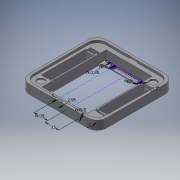
# Autodesk Inventor part: Bauteil1
Saved by Autodesk Inventor 2016 SP2 (Build 200236200, 236)
## iProperties
Created: 2018-06-26
Part Number: Bauteil1
Material: Generisch
Document SubType Name: Modeling
Designer: Nils
Density: 1 g/cm^3
Appearance: Vorgabe
Author: Nils
Autodesk Inventor part; units mm, degrees
ref_plane "YZ Plane" through (0, 0, 0) normal (1, 0, 0) x (0, 1, 0)
ref_plane "XZ Plane" through (0, 0, 0) normal (0, 1, 0) x (-1, 0, 0)
ref_plane "XY Plane" through (0, 0, 0) normal (0, 0, 1) x (1, 0, 0)
sketch "Skizze1" plane through (0, 0, 0) normal (0, 0, 1) x (1, 0, 0)
  line L0 (0, 0) -> (50.3, 0)
  line L1 (50.3, 0) -> (50.3, 70.3)
  line L2 (50.3, 70.3) -> (0, 70.3)
  line L3 (0, 70.3) -> (0, 0)
  line L4 (-15, 75.3) -> (65.3, 75.3)
  line L5 (65.3, 75.3) -> (65.3, -5)
  line L6 (65.3, -5) -> (-15, -5)
  line L7 (-15, -5) -> (-15, 75.3)
  line L8 (-11.7, 59.3) -> (-1.2, 59.3)
  line L9 (-1.2, 59.3) -> (-1.2, 11)
  line L10 (-1.2, 11) -> (-11.7, 11)
  line L11 (-11.7, 11) -> (-11.7, 59.3)
  line L12 (51.5, 59.3) -> (62, 59.3)
  line L13 (62, 59.3) -> (62, 11)
  line L14 (62, 11) -> (51.5, 11)
  line L15 (51.5, 11) -> (51.5, 59.3)
  line L16 (-6.45, 59.3) -> (-6.45, 75.3) construction
  line L17 (-6.45, 11) -> (-6.45, -5) construction
  line L18 (56.75, 59.3) -> (56.75, 75.3) construction
  line L19 (56.75, 11) -> (56.75, -5) construction
  line L20 (-11.7, 35.15) -> (-15, 35.15) construction
  line L21 (62, 35.15) -> (65.3, 35.15) construction
  line L22 (-8.4023, 11) -> (-1.7, 13)
  line L23 (-1.7, 13) -> (-4.95, 14.8)
  line L24 (-4.95, 14.8) -> (-7.95, 14.8)
  line L25 (-7.95, 14.8) -> (-7.95, 14)
  line L26 (-7.95, 14) -> (-5.1567, 14)
  line L27 (-5.1567, 14) -> (-3.7526, 13.2223)
  line L28 (-3.7526, 13.2223) -> (-11.2, 11)
  line L29 (58.25, 55.5) -> (55.25, 55.5)
  line L30 (55.25, 55.5) -> (55.25, 56.3)
  line L31 (55.25, 56.3) -> (58.0433, 56.3)
  line L32 (61.5, 57.3) -> (54.7977, 59.3)
  line L33 (59.4474, 57.0777) -> (52, 59.3)
  line L34 (58.0433, 56.3) -> (59.4474, 57.0777)
  line L35 (58.25, 55.5) -> (61.5, 57.3)
  line L36 (-10.7, 60.9) -> (-2.2, 60.9)
  line L37 (-2.2, 60.9) -> (-2.2, 63.9)
  line L38 (-2.2, 63.9) -> (-10.7, 63.9)
  line L39 (-10.7, 63.9) -> (-10.7, 60.9)
  line L40 (61, 6.4) -> (52.5, 6.4)
  line L41 (52.5, 6.4) -> (52.5, 9.4)
  line L42 (52.5, 9.4) -> (61, 9.4)
  line L43 (61, 9.4) -> (61, 6.4)
  dimension "d0" = 50.3
  dimension "d1" = 70.3
  dimension "d2" = 5
  dimension "d3" = 5
  dimension "d4" = 10.5
  dimension "d5" = 10.5
  dimension "d6" = 48.3
  dimension "d7" = 48.3
  dimension "d8" = 1.2
  dimension "d9" = 1.2
  dimension "d11" = 0.8
  dimension "d12" = 0.8
  dimension "d13" = 0.8
  dimension "d14" = 3
  dimension "d15" = 3.75
  dimension "d16" = 2
  dimension "d17" = 3
  dimension "d18" = 0.5
  dimension "d19" = 0.5
  dimension "d20" = 0.8
  dimension "d22" = 0.5
  dimension "d23" = 3
  dimension "d26" = 3.75
  dimension "d27" = 2
  dimension "d28" = 0.5
  dimension "d30" = 3
  dimension "d31" = 0.8
  dimension "d32" = 0.8
  dimension "d33" = 1.6
  dimension "d34" = 1
  dimension "d35" = 1
  dimension "d36" = 3
  dimension "d37" = 3
  dimension "d38" = 1
  dimension "d39" = 1
  dimension "d40" = 1.6
  constraints: 88 end point, 17 parallel, 13 perpendicular, 10 point on line, 8 midpoint, 7 horizontal, 4 equal length
  measures "d0" distance of L2.end L1.end
  measures "d1" distance of L1.end L0.end
  measures "d2" distance between parallel lines of L2 L4
  measures "d3" distance between parallel lines of L6 L0
  measures "d4" distance between parallel lines of L9 L11
  measures "d5" distance of L12.start L12.end
  measures "d6" distance between parallel lines of L10 L8
  measures "d7" distance of L12.end L13.end
  measures "d8" distance between parallel lines of L3 L9
  measures "d9" distance between parallel lines of L15 L1
  measures "d11" distance between parallel lines of L22 L28
  measures "d12" distance between parallel lines of L23 L27
  measures "d13" distance between parallel lines of L26 L24
  measures "d14" distance of L23.end L24.end
  measures "d15" distance between parallel lines of L11 L25
  measures "d16" distance from line of L10 L22.end
  measures "d17" distance between parallel lines of L10 L26
  measures "d18" distance of L28.end L10.end
  measures "d19" distance from line of L9 L22.end
  measures "d20" distance between parallel lines of L29 L31
  measures "d22" distance from line of L13 L32.start
  measures "d23" distance of L29.start L29.end
  measures "d26" distance between parallel lines of L15 L30
  measures "d27" distance from line of L12 L32.start
  measures "d28" distance of L12.start L33.end
  measures "d30" distance between parallel lines of L12 L31
  measures "d31" distance between parallel lines of L35 L34
  measures "d32" distance between parallel lines of L32 L33
  measures "d33" distance between parallel lines of L8 L36
  measures "d34" distance between parallel lines of L39 L11
  measures "d35" distance between parallel lines of L9 L37
  measures "d36" distance between parallel lines of L36 L38
  measures "d37" distance of L40.end L41.end
  measures "d38" distance between parallel lines of L13 L43
  measures "d39" distance between parallel lines of L41 L15
  measures "d40" distance between parallel lines of L42 L14
extrude "Extrusion1" add sketch "Skizze1" along normal blind 10 contours L4 L5 L6 L7 | L28 L27 L26 L25 L24 L23 L22 L10 | L12 L32 L35 L29 L30 L31 L34 L33
sketch "Skizze2" plane through (0, 0, 0) normal (0, 0, -1) x (-1, 0, 0)
  line L0 (-65.3, 75.3) -> (15, 75.3) projected
  line L1 (15, 75.3) -> (15, -5) projected
  line L2 (-65.3, 75.3) -> (15, 75.3)
  line L3 (15, 75.3) -> (15, -5)
  line L4 (15, -5) -> (-65.3, -5)
  line L5 (-65.3, -5) -> (-65.3, 75.3)
  line L6 (0, 70.3) -> (0, 0) projected
  line L7 (-48.3, 64.65) -> (-2, 64.65)
  line L8 (0, 62.65) -> (0, 7.65)
  line L9 (-2, 5.65) -> (-48.3, 5.65)
  line L10 (-50.3, 7.65) -> (-50.3, 62.65)
  line L11 (-50.3, 70.3) -> (0, 70.3) projected
  line L12 (-50.3, 0) -> (-50.3, 70.3) construction
  arc A0 (-48.3, 64.65) -> (-50.3, 62.65) centre (-48.3, 62.65) ccw
  arc A1 (0, 62.65) -> (-2, 64.65) centre (-2, 62.65) ccw
  arc A2 (-50.3, 7.65) -> (-48.3, 5.65) centre (-48.3, 7.65) ccw
  arc A3 (-2, 5.65) -> (0, 7.65) centre (-2, 7.65) ccw
  line L13 (15, 35.15) -> (-65.3, 35.15) construction
  line L14 (-65.3, -5) -> (-65.3, 75.3) construction
  line L15 (-50.3, 0) -> (0, 0) construction
  point P0 (-50.3, 64.65)
  point P1 (0, 5.65)
  dimension "d44" = 59
  dimension "d45" = 2
  dimension "d147" = 29.5
  constraints: 18 end point, 8 point on circle, 8 tangent, 6 point on line, 4 centre point, 4 parallel, 3 equal radius, 2 horizontal, 2 midpoint, 2 perpendicular
  measures "d44" distance between parallel lines of L9 L7
  measures "d45" radius of A0
  measures "d147" distance between parallel lines of L7 L13
extrude "Extrusion2" add sketch "Skizze2" along normal blind 0.8
sketch "Skizze7" plane through (0, 0, 10) normal (0, 0, 1) x (1, 0, 0)
  circle A0 centre (-6, 5) radius 4.075
  circle A1 centre (56.3, 65.3) radius 4.075
  line L0 (0, 0) -> (0, 70.3) projected
  line L1 (-1.2, 11) -> (-8.4023, 11) projected
  line L2 (50.3, 70.3) -> (50.3, 0) projected
  line L3 (54.7977, 59.3) -> (62, 59.3) projected
  dimension "d80" = 8.15
  dimension "d81" = 8.15
  dimension "d82" = 6
  dimension "d83" = 6
  dimension "d84" = 6
  dimension "d85" = 6
  constraints: 2 centre point
  measures "d80" diameter of A0
  measures "d81" diameter of A1
  measures "d82" distance from line of L0 A0.centre
  measures "d83" distance from line of L1 A0.centre
  measures "d84" distance from line of L2 A1.centre
  measures "d85" distance from line of L3 A1.centre
extrude "Extrusion7" cut sketch "Skizze7" against normal blind 1.4
sketch "Skizze8" plane through (55.25, 55.5, 10) normal (0, -1, 0) x (1, 0, 0)
  line L0 (-3.75, -10) -> (-3.75, 0) projected
  line L1 (6.75, -10) -> (-3.75, -10)
  line L2 (-3.75, -10) -> (-3.75, -7)
  line L3 (-3.75, -7) -> (6.75, -7)
  line L4 (6.75, -7) -> (6.75, -10)
  line L5 (-3.75, 0) -> (6.75, 0)
  line L6 (6.75, 0) -> (6.75, -3)
  line L7 (6.75, -3) -> (-3.75, -3)
  line L8 (-3.75, -3) -> (-3.75, 0)
  point P0 (-55.25, -10)
  dimension "d88" = 3
  dimension "d89" = 3
  constraints: 16 end point, 4 parallel, 2 horizontal, 2 perpendicular, 2 point on line
  measures "d88" distance of L3.end L1.start
  measures "d89" distance between parallel lines of L5 L7
extrude "Extrusion8" cut sketch "Skizze8" against normal blind 3.8
sketch "Skizze9" plane through (-7.95, 14.8, 10) normal (0, 1, 0) x (1, 0, 0)
  line L0 (-3.75, 10) -> (-3.75, 0) projected
  line L1 (6.75, 10) -> (-3.75, 10)
  line L2 (-3.75, 10) -> (-3.75, 7)
  line L3 (-3.75, 7) -> (6.75, 7)
  line L4 (6.75, 7) -> (6.75, 10)
  line L5 (6.75, 0) -> (-3.75, 0)
  line L6 (-3.75, 0) -> (-3.75, 3)
  line L7 (-3.75, 3) -> (6.75, 3)
  line L8 (6.75, 3) -> (6.75, 0)
  point P0 (7.95, 10)
  dimension "d92" = 3
  dimension "d93" = 3
  constraints: 16 end point, 4 parallel, 2 horizontal, 2 perpendicular, 2 point on line
  measures "d92" distance of L5.end L6.end
  measures "d93" distance between parallel lines of L1 L3
extrude "Extrusion9" cut sketch "Skizze9" against normal blind 3.8
sketch "Skizze10" plane through (0, 0, 10) normal (0, 0, 1) x (1, 0, 0)
  line L0 (52.5, 9.4) -> (61, 9.4) projected
  line L1 (62, 11) -> (51.5, 11) projected
  line L2 (52.5, 9.4) -> (61, 9.4)
  line L3 (61, 9.4) -> (61, 11)
  line L4 (61, 11) -> (52.5, 11)
  line L5 (52.5, 11) -> (52.5, 9.4)
  line L6 (52.5, 6.4) -> (52.5, 9.4) projected
  line L7 (50.3, 70.3) -> (50.3, 0) projected
  line L8 (52.5, 6.9) -> (50.3, 6.9)
  line L9 (50.3, 6.9) -> (50.3, 8.9)
  line L10 (50.3, 8.9) -> (52.5, 8.9)
  line L11 (52.5, 8.9) -> (52.5, 6.9)
  line L12 (51.5, 11) -> (51.5, 59.3) projected
  line L13 (51.5, 58.8) -> (50.3, 58.8)
  line L14 (50.3, 58.8) -> (50.3, 56.8)
  line L15 (50.3, 56.8) -> (51.5, 56.8)
  line L16 (51.5, 56.8) -> (51.5, 58.8)
  line L17 (51.5, 59.3) -> (62, 59.3) projected
  line L18 (-1.2, 59.3) -> (-1.2, 11) projected
  line L19 (-1.2, 11.5) -> (0, 11.5)
  line L20 (0, 11.5) -> (0, 13.5)
  line L21 (0, 13.5) -> (-1.2, 13.5)
  line L22 (-1.2, 13.5) -> (-1.2, 11.5)
  line L23 (-1.2, 11) -> (-11.7, 11) projected
  line L24 (0, 0) -> (0, 70.3) construction
  line L25 (-2.2, 60.9) -> (-10.7, 60.9) projected
  line L26 (-10.7, 60.9) -> (-2.2, 60.9)
  line L27 (-2.2, 60.9) -> (-2.2, 59.3)
  line L28 (-2.2, 59.3) -> (-10.7, 59.3)
  line L29 (-10.7, 59.3) -> (-10.7, 60.9)
  line L30 (-2.2, 63.9) -> (-2.2, 60.9) projected
  line L31 (-2.2, 63.4) -> (0, 63.4)
  line L32 (0, 63.4) -> (0, 61.4)
  line L33 (0, 61.4) -> (-2.2, 61.4)
  line L34 (-2.2, 61.4) -> (-2.2, 63.4)
  dimension "d96" = 8.5
  dimension "d97" = 0.5
  dimension "d98" = 0.5
  dimension "d99" = 2
  dimension "d100" = 0.5
  dimension "d101" = 2
  dimension "d102" = 0.5
  dimension "d103" = 1.6
  dimension "d104" = 8.5
  dimension "d105" = 2
  dimension "d106" = 0.5
  constraints: 48 end point, 12 parallel, 9 point on line, 6 horizontal, 6 perpendicular
  measures "d96" distance between parallel lines of L3 L5
  measures "d97" distance between parallel lines of L0 L10
  measures "d98" distance from line of L6.start L8
  measures "d99" distance of L14.end L13.end
  measures "d100" distance between parallel lines of L17 L13
  measures "d101" distance of L20.end L19.end
  measures "d102" distance between parallel lines of L19 L23
  measures "d103" distance of L28.end L25.end
  measures "d104" distance between parallel lines of L29 L27
  measures "d105" distance between parallel lines of L33 L31
  measures "d106" distance between parallel lines of L33 L25
extrude "Extrusion10" cut sketch "Skizze10" against normal blind 1.5 contours L5 L1 L3 L0 | L6 L8 L7 L10 | L15 L7 L13 L12 | L21 L20 L19 L18 | L27 L28 L29 L25 | L31 L32 L33 L30
sketch "Skizze12" plane through (0, 0, 10) normal (0, 0, 1) x (1, 0, 0)
  line L0 (-15, -5) -> (65.3, -5)
  line L1 (65.3, -5) -> (65.3, 75.3)
  line L2 (65.3, 75.3) -> (-15, 75.3)
  line L3 (-15, 75.3) -> (-15, -5)
  line L4 (-15, 75.3) -> (-15, -5) projected
  line L5 (50.3, 56.8) -> (50.3, 8.9) projected
  line L6 (48.3, 5.65) -> (2, 5.65) projected
  line L7 (2, 64.65) -> (48.3, 64.65) projected
  line L8 (0, 0) -> (0, 11.5) projected
  line L9 (-11.7, 59.3) -> (-11.7, 11) projected
  line L10 (0, 0) -> (50.3, 0) projected
  line L11 (62, 59.3) -> (62, 11) projected
  line L12 (0, 70.3) -> (50.3, 70.3) projected
  line L13 (-16.9, 77.2) -> (67.2, 77.2)
  line L14 (67.2, 77.2) -> (67.2, -6.9)
  line L15 (67.2, -6.9) -> (-16.9, -6.9)
  line L16 (-16.9, -6.9) -> (-16.9, 77.2)
  line L17 (-14.4, 74.7) -> (64.7, 74.7)
  line L18 (64.7, 74.7) -> (64.7, -4.4)
  line L19 (64.7, -4.4) -> (-14.4, -4.4)
  line L20 (-14.4, -4.4) -> (-14.4, 74.7)
  point P0 (35.15, 0)
  point P1 (45.3, 70.3)
  dimension "d124" = 1.9
  dimension "d125" = 0.6
  constraints: 24 end point, 6 parallel, 3 perpendicular, 1 horizontal, 6 other
  measures "d124" distance between parallel lines of L2 L13
  measures "d125" distance between parallel lines of L2 L17
extrude "Extrusion12" add sketch "Skizze12" along normal blind 2.6 contours L3 L2 L1 L0 | L13 L14 L15 L16
sketch "Skizze13" plane through (-14.4, -4.4, 10) normal (0, 1, 0) x (1, 0, 0)
  line L0 (64.7, 10) -> (64.7, 0) projected
  line L1 (64.7, 0) -> (59.5, 0)
  line L2 (59.5, 0) -> (59.5, -1)
  line L3 (59.5, -1) -> (64.7, -1)
  line L4 (64.7, -1) -> (64.7, 0)
  line L5 (14.4, 10) -> (14.4, 0) projected
  line L6 (14.4, 0) -> (19.6, 0)
  line L7 (19.6, 0) -> (19.6, -1)
  line L8 (19.6, -1) -> (14.4, -1)
  line L9 (14.4, -1) -> (14.4, 0)
  dimension "d126" = 5.2
  dimension "d127" = 1
  dimension "d128" = 5.2
  dimension "d129" = 1
  constraints: 16 end point, 4 parallel, 2 horizontal, 2 perpendicular
  measures "d126" distance of L3.end L2.end
  measures "d127" distance of L2.end L1.end
  measures "d128" distance of L7.end L8.end
  measures "d129" distance of L6.end L7.end
extrude "Extrusion13" cut sketch "Skizze13" against normal blind 1.2
sketch "Skizze14" plane through (-14.4, 74.7, 10) normal (0, -1, 0) x (1, 0, 0)
  line L0 (79.1, 0) -> (0, 0) projected
  line L1 (39.55, 0) -> (43.65, 0)
  line L2 (43.65, 0) -> (43.65, 1)
  line L3 (0, 2.6) -> (79.1, 2.6) projected
  line L4 (43.65, 1) -> (35.45, 1)
  line L5 (35.45, 1) -> (35.45, 0)
  line L6 (-2.5, 0) -> (81.6, 0) projected
  line L7 (35.45, 0) -> (39.55, 0)
  point P0 (14.4, -10)
  dimension "d132" = 4.1
  dimension "d133" = 1
  dimension "d134" = 8.2
  constraints: 10 end point, 2 perpendicular, 2 point on line, 1 collinear, 1 midpoint, 1 parallel
  measures "d132" distance of L1.start L1.end
  measures "d133" distance of L1.end L2.end
  measures "d134" distance of L2.end L4.end
extrude "Extrusion14" cut sketch "Skizze14" against normal blind 1.2
sketch "Skizze15" plane through (0, 0, 10) normal (0, 0, -1) x (-1, 0, 0)
  line L0 (-67.2, 77.2) -> (-67.2, -6.9) projected
  line L1 (-67.2, -6.9) -> (16.9, -6.9) projected
  line L2 (16.9, -6.9) -> (16.9, 77.2) projected
  line L3 (16.9, 77.2) -> (-67.2, 77.2) projected
  line L4 (15, 75.3) -> (-65.3, 75.3) projected
  line L5 (15, 75.3) -> (15, -5) projected
  line L6 (-65.3, 75.3) -> (15, 75.3)
  line L7 (15, 75.3) -> (15, -5)
  line L8 (15, -5) -> (-65.3, -5)
  line L9 (-65.3, -5) -> (-65.3, 75.3)
  point P0 (0, 0)
  constraints: 8 end point, 2 parallel, 1 horizontal, 1 perpendicular
extrude "Extrusion15" add sketch "Skizze15" along normal blind 10.8
fillet "Rundung1" radius 10 8 edges at (64.7, -4.4, 11.3) (-14.4, -4.4, 11.3) (64.7, 74.7, 11.3) (-14.4, 74.7, 11.3) (67.2, 77.2, 5.9) (67.2, -6.9, 5.9) (-16.9, -6.9, 5.9) (-16.9, 77.2, 5.9)
chamfer "Fase3" distance 5.3 angle 35 8 edges at (-13.9711, -3.9711, -0.8) (25.15, -6.9, -0.8) (64.2711, -3.9711, -0.8) (67.2, 35.15, -0.8) (64.2711, 74.2711, -0.8) (25.15, 77.2, -0.8) (-13.9711, 74.2711, -0.8) (-16.9, 35.15, -0.8) measured on face at (-16.4, 35.15, -0.8) measured on face at (63.9175, 73.9175, -0.8) measured on face at (66.7, 35.15, -0.8) measured on face at (-13.6175, 73.9175, -0.8) measured on face at (25.15, -6.4, -0.8) measured on face at (63.9175, -3.6175, -0.8) measured on face at (-13.6175, -3.6175, -0.8) measured on face at (25.15, 76.7, -0.8)
sketch "Skizze17" plane through (0, 0, 0) normal (0, 0, 1) x (1, 0, 0)
  line L0 (0, 0) -> (0, 11.5) projected
  line L1 (50.3, 6.9) -> (50.3, 0) projected
  line L2 (0, 0) -> (50.3, 0)
  line L3 (50.3, 0) -> (50.3, 1.4)
  line L4 (50.3, 1.4) -> (0, 1.4)
  line L5 (0, 1.4) -> (0, 0)
  line L6 (0, 70.3) -> (0, 62.65) projected
  line L7 (50.3, 62.65) -> (50.3, 70.3) projected
  line L8 (0, 70.3) -> (50.3, 70.3)
  line L9 (50.3, 70.3) -> (50.3, 69)
  line L10 (50.3, 69) -> (0, 69)
  line L11 (0, 69) -> (0, 70.3)
  line L12 (50.3, 2.95) -> (0, 2.95) construction
  line L13 (50.3, 67.35) -> (0, 67.35) construction
  line L14 (50.3, 0) -> (0, 0) construction
  line L15 (40.15, 0) -> (40.15, 70.3) construction
  line L16 (50.3, 70.3) -> (0, 70.3) construction
  line L17 (10.15, 0) -> (10.15, 70.3) construction
  line L18 (25.15, 0) -> (25.15, 70.3) construction
  circle A0 centre (10.15, 2.95) radius 2.5
  circle A1 centre (10.15, 2.95) radius 1.5
  circle A2 centre (40.15, 2.95) radius 2.5
  circle A3 centre (40.15, 2.95) radius 1.5
  circle A4 centre (40.15, 67.35) radius 2.5
  circle A5 centre (40.15, 67.35) radius 1.5
  circle A6 centre (10.15, 67.35) radius 2.5
  circle A7 centre (10.15, 67.35) radius 1.5
  dimension "d150" = 1.4
  dimension "d151" = 1.3
  dimension "d152" = 5
  dimension "d153" = 3
  dimension "d154" = 3
  dimension "d155" = 5
  dimension "d156" = 3
  dimension "d157" = 5
  dimension "d158" = 3
  dimension "d159" = 5
  dimension "d160" = 2.95
  dimension "d161" = 2.95
  dimension "d162" = 15
  dimension "d163" = 15
  constraints: 26 end point, 18 point on line, 8 centre point, 5 parallel, 5 perpendicular, 4 coincident, 2 horizontal, 2 midpoint
  measures "d150" distance of L3.end L2.end
  measures "d151" distance of L8.end L9.end
  measures "d152" diameter of A0
  measures "d153" diameter of A1
  measures "d154" diameter of A7
  measures "d155" diameter of A6
  measures "d156" diameter of A3
  measures "d157" diameter of A2
  measures "d158" diameter of A5
  measures "d159" diameter of A4
  measures "d160" distance between parallel lines of L12 L2
  measures "d161" distance between parallel lines of L13 L8
  measures "d162" distance between parallel lines of L15 L18
  measures "d163" distance between parallel lines of L17 L18
equation "\"d3\" = d2"
equation "\"d5\" = d4"
equation "\"d7\" = d6"
equation "\"d22\" = d21"
equation "\"d35\" = d34"
equation "\"d39\" = d38"
equation "\"d147\" = 0.5 * d44"
equation "\"d81\" = d80"
equation "\"d83\" = d82"
equation "\"d84\" = d82"
equation "\"d85\" = d84"
equation "\"d89\" = d88"
equation "\"d93\" = d92"
equation "\"d21\" = 0.5"
